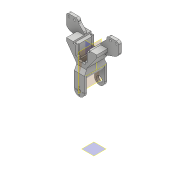
# Autodesk Inventor part: core_structure
Saved by Autodesk Inventor 2018 (Build 220112000, 112)
## iProperties
Created: 2018-02-12
Part Number: core_structure
Material: Generic
Document SubType Name: Modeling
Designer: Bardo91
Density: 1 g/cm^3
Appearance: Default
Author: Bardo91
Autodesk Inventor part; units mm, degrees
ref_plane "YZ Plane" through (0, 0, 0) normal (1, 0, 0) x (0, 1, 0)
ref_plane "XZ Plane" through (0, 0, 0) normal (0, 1, 0) x (-1, 0, 0)
ref_plane "XY Plane" through (0, 0, 0) normal (0, 0, 1) x (1, 0, 0)
sketch "Sketch1" plane through (0, 0, 0) normal (0, 0, 1) x (1, 0, 0)
  line L0 (0, 0) -> (18, 0)
  line L1 (18, 0) -> (18, 32)
  line L2 (18, 32) -> (0, 32)
  line L3 (0, 32) -> (0, 0)
  dimension "d0" = 18
  dimension "d1" = 32
  constraints: 8 end point, 2 perpendicular, 1 horizontal, 1 vertical
  measures "d0" distance of L0.start L0.end
  measures "d1" distance of L0.end L1.end
extrude "base" add sketch "Sketch1" along normal blind 25
sketch "Sketch2" plane through (0, 0, 25) normal (0, 0, 1) x (1, 0, 0)
  line L0 (18, 32) -> (0, 32) projected
  line L1 (9, 32) -> (9, 0)
  line L2 (9, 16) -> (9, 27.5)
  line L3 (9, 16) -> (20.5, 16) construction
  line L4 (9, 27.5) -> (15.25, 27.5)
  line L5 (15.25, 27.5) -> (15.25, 4.5)
  line L6 (15.25, 4.5) -> (2.75, 4.5)
  line L7 (2.75, 4.5) -> (2.75, 27.5)
  line L8 (2.75, 27.5) -> (9, 27.5)
  line L9 (0, 0) -> (18, 0) projected
  dimension "d4" = 11.5
  dimension "d5" = 90
  dimension "d6" = 6.25
  dimension "d7" = 23
  dimension "d8" = 12.5
  constraints: 16 end point, 6 perpendicular, 3 midpoint, 1 collinear, 1 horizontal, 1 point on line, 1 vertical
  measures "d4" distance of L2.start L2.end
  measures "d5" angle of L3 L2
  measures "d6" distance of L2.end L4.end
  measures "d7" distance of L4.end L5.end
  measures "d8" distance of L5.end L6.end
extrude "servo_place" cut sketch "Sketch2" against normal blind 18
sketch "Sketch3" plane through (0, 0, 25) normal (0, 0, 1) x (1, 0, 0)
  line L0 (2.75, 27.5) -> (15.25, 27.5) projected
  line L1 (9, 27.5) -> (9, 30.3)
  circle A0 centre (9, 30.3) radius 1
  line L2 (15.25, 4.5) -> (2.75, 4.5) projected
  line L3 (9, 4.5) -> (9, 1.7)
  circle A1 centre (9, 1.7) radius 1
  point P0 (0, 0)
  dimension "d11" = 2.8
  dimension "d12" = 2
  dimension "d13" = 2.8
  dimension "d14" = 2
  constraints: 4 end point, 2 centre point, 2 coincident, 2 midpoint, 2 vertical
  measures "d11" distance of L1.start L1.end
  measures "d12" diameter of A0
  measures "d13" distance of L3.start L3.end
  measures "d14" diameter of A1
extrude "screws_servo" cut sketch "Sketch3" against normal through all
ref_plane "Work Plane1" through (9, 22, -120) normal (0, 0, -1) x (-1, 0, 0)
sketch "Sketch6" plane through (0, 0, 25) normal (0, 0, 1) x (1, 0, 0)
  line L0 (0, 32) -> (0, 0) projected
  line L1 (2.75, 27.5) -> (15.25, 27.5) projected
  line L2 (0, 32) -> (2.75, 32)
  line L3 (2.75, 32) -> (2.75, 27.5)
  line L4 (2.75, 27.5) -> (0, 27.5)
  line L5 (0, 27.5) -> (0, 32)
  line L6 (18, 32) -> (15.2563, 32)
  line L7 (15.2563, 32) -> (15.2563, 27.5)
  line L8 (15.2563, 27.5) -> (18, 27.5)
  line L9 (18, 27.5) -> (18, 32)
  line L10 (15.25, 27.5) -> (15.25, 4.5) projected
  line L11 (18, 0) -> (15.25, 0)
  line L12 (15.25, 0) -> (15.25, 4.5)
  line L13 (15.25, 4.5) -> (18, 4.5)
  line L14 (18, 4.5) -> (18, 0)
  line L15 (0, 0) -> (2.75, 0)
  line L16 (2.75, 0) -> (2.75, 4.5)
  line L17 (2.75, 4.5) -> (0, 4.5)
  line L18 (0, 4.5) -> (0, 0)
  constraints: 32 end point, 8 parallel, 4 horizontal, 4 perpendicular, 4 point on line
extrude "pilars_top" add sketch "Sketch6" along normal blind 20
sketch "Sketch9" plane through (0, 0, 45) normal (0, 0, 1) x (1, 0, 0)
  line L0 (0, 32) -> (0, 0) projected
  line L1 (18, 0) -> (18, 32) projected
  line L2 (0, 32) -> (18, 32)
  line L3 (18, 32) -> (18, 0)
  line L4 (18, 0) -> (0, 0)
  line L5 (0, 0) -> (0, 32)
  line L6 (18, 32) -> (36, 32)
  line L7 (36, 32) -> (36, 0)
  line L8 (36, 0) -> (18, 0)
  line L9 (0, 32) -> (-18, 32)
  line L10 (-18, 32) -> (-18, 0)
  line L11 (-18, 0) -> (0, 0)
  point P0 (0, 22)
  point P1 (18, 22)
  dimension "d39" = 18
  dimension "d40" = 18
  constraints: 20 end point, 5 perpendicular, 3 parallel, 1 horizontal, 1 point on line, 1 vertical
  measures "d39" distance of L1.end L6.end
  measures "d40" distance of L0.start L9.end
extrude "base_top" add sketch "Sketch9" along normal blind 5
sketch "Sketch10" plane through (0, 0, 50) normal (0, 0, 1) x (1, 0, 0)
  line L0 (18, 32) -> (0, 32) projected
  line L1 (15.293, 32) -> (15.293, 0)
  line L2 (15.25, 27.5) -> (15.25, 4.5) projected
  line L3 (15.2563, 27.5) -> (15.2563, 32) projected
  line L4 (15.2563, 32) -> (2.7563, 32)
  line L5 (36, 32) -> (-18, 32) projected
  line L6 (2.7563, 32) -> (2.7563, 0)
  line L7 (0, 0) -> (18, 0) projected
  line L8 (15.293, 0) -> (2.7563, 0)
  dimension "d100" = 12.5
  constraints: 8 end point, 3 point on line, 1 collinear, 1 parallel, 1 perpendicular
  measures "d100" distance of L3.end L4.end
extrude "screw_hole" cut sketch "Sketch10" against normal blind 5
ref_plane "Work Plane2" through (0, 0, 10) normal (0, 0, -1) x (-1, 0, 0)
sketch "Sketch12" plane through (0, 0, 10) normal (0, 0, -1) x (-1, 0, 0)
  line L0 (0, 0) -> (-18, 0) projected
  line L1 (-18, 0) -> (-18, -4)
  line L2 (-18, -4) -> (0, -4)
  line L3 (0, -4) -> (0, 0)
  line L4 (0, 0) -> (0, -4)
  line L5 (0, 0) -> (-18, 0)
  line L6 (-18, 32) -> (0, 32) projected
  line L7 (-18, 32) -> (0, 32)
  line L8 (0, 32) -> (0, 36)
  line L9 (0, 36) -> (-18, 36)
  line L10 (-18, 36) -> (-18, 32)
  dimension "d64" = 4
  dimension "d65" = 4
  constraints: 18 end point, 4 perpendicular, 3 collinear, 2 point on line, 1 vertical
  measures "d64" distance of L0.end L1.end
  measures "d65" distance of L6.end L8.end
extrude "connector_prev_servo" add sketch "Sketch12" along normal blind 36
chamfer "Chamfer2" distance 8 distance2 4 1 edges at (9, 32, 10) measured on face at (9, 32, 10.5)
fillet "Fillet3" radius 9 4 edges at (18, 34, -26) (0, 34, -26) (0, -2, -26) (18, -2, -26)
sketch "Sketch13" plane through (0, -4, 10) normal (0, -1, 0) x (1, 0, 0)
  arc A0 (0, -27) -> (18, -27) centre (9, -27) ccw projected
  circle A1 centre (9, -27) radius 2.75
  line L0 (9, -27) -> (15, -27)
  circle A2 centre (15, -27) radius 1
  circle A3 centre (9, -21) radius 1
  circle A4 centre (3, -27) radius 1
  circle A5 centre (9, -33) radius 1
  point P0 (0, -10)
  dimension "d72" = 5.5
  dimension "d73" = 6
  dimension "d74" = 2
  dimension "d77" = 360
  constraints: 5 centre point, 2 coincident, 2 end point, 1 horizontal, 9 other
  measures "d72" diameter of A1
  measures "d73" distance of L0.start L0.end
  measures "d74" diameter of A2
extrude "screw_holes" cut sketch "Sketch13" against normal up to surface (4 mm away)
fillet "Fillet4" radius 9 2 edges at (18, 16, 0) (0, 16, 0)
sketch "Sketch14" plane through (0, 36, 10) normal (0, 1, 0) x (1, 0, 0)
  arc A0 (18, 27) -> (0, 27) centre (9, 27) ccw projected
  circle A1 centre (9, 27) radius 5.25
  point P0 (0, 10)
  dimension "d82" = 10.5
  constraints: 1 centre point, 1 coincident
  measures "d82" diameter of A1
extrude "Extrusion14" cut sketch "Sketch14" against normal up to next
sketch "Sketch16" plane through (2.75, 0, 25) normal (0, -1, 0) x (1, 0, 0)
  line L0 (12.5063, 20) -> (15.25, 20) projected
  line L1 (15.25, 20) -> (33.25, 20)
  line L2 (15.25, 20) -> (15.25, -5)
  line L3 (15.25, -7) -> (15.25, 20) projected
  line L4 (15.25, -5) -> (33.25, 20)
  point P0 (-2.75, -25)
  dimension "d95" = 25
  constraints: 6 end point, 1 horizontal, 1 point on line
  measures "d95" distance of L0.end L2.end
extrude "Extrusion16" add sketch "Sketch16" against normal blind 4.6
ref_plane "Work Plane3" through (2.75, 16, 25) normal (0, 1, 0) x (1, 0, 0)
ref_plane "Work Plane4" through (9, -4, -17) normal (1, 0, 0) x (0, 0, -1)
mirror "Mirror1" about plane through (2.75, 16, 25) normal (0, 1, 0) of "Extrusion16"
mirror "Mirror2" about plane through (9, -4, -17) normal (1, 0, 0) of "Extrusion16", "Mirror1"
sketch "Sketch18" plane through (2.75, 0, 25) normal (0, -1, 0) x (1, 0, 0)
  line L0 (12.5, 0) -> (0, 0) projected
  line L1 (6.25, 0) -> (6.25, 5)
  line L2 (6.25, 5) -> (-3.75, 5)
  line L3 (-3.75, 5) -> (-3.75, 25)
  line L4 (-20.75, 25) -> (0.0063, 25) projected
  line L5 (-3.75, 25) -> (16.25, 25)
  line L6 (16.25, 25) -> (16.25, 5)
  line L7 (16.25, 5) -> (6.25, 5)
  point P0 (-2.75, -25)
  dimension "d105" = 5
  dimension "d106" = 10
  dimension "d107" = 20
  constraints: 12 end point, 5 perpendicular, 2 point on line, 1 midpoint, 1 vertical
  measures "d105" distance of L1.start L1.end
  measures "d106" distance of L1.end L2.end
  measures "d107" distance of L3.end L5.end
extrude "Extrusion18" cut sketch "Sketch18" against normal through all
sketch "Sketch19" plane through (0, 0, 50) normal (0, 0, 1) x (1, 0, 0)
  line L0 (-1, 0) -> (-1, 32) projected
  line L1 (-1, 32) -> (-6, 32)
  line L2 (0, 32) -> (-18, 32) projected
  line L3 (-6, 32) -> (-6, 0)
  line L4 (-6, 0) -> (24, 0)
  line L5 (24, 0) -> (24, 32)
  line L6 (24, 32) -> (-1, 32)
  point P0 (0, 0)
  dimension "d110" = 5
  dimension "d111" = 30
  constraints: 10 end point, 4 perpendicular, 2 point on line
  measures "d110" distance of L0.end L1.end
  measures "d111" distance of L3.end L4.end
extrude "Extrusion19" cut sketch "Sketch19" against normal blind 3
sketch "Sketch20" plane through (0, 0, 47) normal (0, 0, 1) x (1, 0, 0)
  line L0 (-6, 32) -> (-1, 32) projected
  line L1 (-6, 32) -> (-3.5, 32)
  line L2 (-3.5, 32) -> (-3.5, 29.5)
  circle A0 centre (-3.5, 29.5) radius 1.4
  point P0 (0, 0)
  dimension "d114" = 2.5
  dimension "d115" = 2.5
  dimension "d116" = 2.8
  constraints: 4 end point, 1 centre point, 1 coincident, 1 midpoint, 1 perpendicular
  measures "d114" distance of L0.start L1.end
  measures "d115" distance of L1.end L2.end
  measures "d116" diameter of A0
extrude "Extrusion20" cut sketch "Sketch20" against normal blind 5
mirror "Mirror3" about plane through (9, -4, -17) normal (1, 0, 0) of "Extrusion20"
mirror "Mirror4" about plane through (2.75, 16, 25) normal (0, 1, 0) of "Extrusion20", "Mirror3"
sketch "Sketch21" plane through (0, 0, 25) normal (0, 0, 1) x (1, 0, 0)
  line L0 (2.75, 4.5) -> (2.75, 27.5) projected
  line L1 (2.75, 16) -> (2.75, 27.75)
  line L2 (2.75, 27.75) -> (15.25, 27.75)
  line L3 (15.25, 27.75) -> (15.25, 4.25)
  line L4 (15.25, 27.5) -> (15.25, 4.5) projected
  line L5 (15.25, 4.25) -> (2.75, 4.25)
  line L6 (2.75, 4.25) -> (2.75, 16)
  point P0 (0, 0)
  dimension "d119" = 11.75
  dimension "d120" = 12.5
  dimension "d121" = 23.5
  dimension "d122" = 12.5
  constraints: 10 end point, 2 collinear, 1 midpoint, 1 perpendicular, 1 point on line
  measures "d119" distance of L1.start L1.end
  measures "d120" distance of L1.end L2.end
  measures "d121" distance of L2.end L3.end
  measures "d122" distance of L3.end L5.end
extrude "Extrusion21" cut sketch "Sketch21" against normal up to surface (18 mm away)
sketch "Sketch22" plane through (2.75, 27.75, 25) normal (0, -1, 0) x (1, 0, 0)
  line L0 (12.5, 0) -> (12.5, -18) projected
  line L1 (0, -18) -> (12.5, -18) projected
  line L2 (12.5, -18) -> (0, -18)
  line L3 (0, -18) -> (0, -11)
  line L4 (0, -11) -> (12.5, -11)
  line L5 (12.5, -11) -> (12.5, -18)
  point P0 (-2.75, -25)
  dimension "d125" = 7
  constraints: 8 end point, 3 perpendicular, 1 collinear
  measures "d125" distance of L1.start L3.end
extrude "Extrusion22" cut sketch "Sketch22" against normal through all
chamfer "Chamfer3" distance 8 distance2 4 1 edges at (9, 0, 10) measured on face at (9, 0, 10.5)
sketch "Sketch23" plane through (18, 27.4, 20) normal (0, -1, 0) x (1, 0, 0)
  line L0 (18, 25) -> (1, 25) projected
  line L1 (18, 25) -> (1, 25)
  line L2 (0, 0) -> (18, 25) projected
  line L3 (18, 25) -> (0, 0)
  line L4 (0, 0) -> (0, 5) projected
  line L5 (0, 0) -> (0, 27)
  line L6 (0, 27) -> (18, 27)
  line L7 (18, 27) -> (18, 25)
  line L8 (-35.987, 24.982) -> (-18, 0)
  line L9 (-18, 0) -> (-36, 25) projected
  line L10 (-18, 0) -> (-18, 27)
  line L11 (-18, 27) -> (-35.987, 27)
  line L12 (-35.987, 27) -> (-35.987, 24.982)
  point P0 (-18, -20)
  dimension "d131" = 27
  dimension "d132" = 27
  constraints: 18 end point, 4 perpendicular, 3 collinear, 2 point on line, 1 horizontal, 1 vertical
  measures "d131" distance of L5.start L5.end
  measures "d132" distance of L8.end L10.end
extrude "Extrusion23" add sketch "Sketch23" along normal up to surface (22.8 mm away)
sketch "Sketch11" plane through (0, 0, 50) normal (0, 0, 1) x (1, 0, 0)
  circle A0 centre (9, 22) radius 6 projected
  line L0 (9, 22) -> (36, 22)
  line L1 (36, 0) -> (36, 32) projected
  line L2 (36, 22) -> (36, 24.5)
  line L3 (36, 24.5) -> (31, 24.5)
  line L4 (31, 24.5) -> (31, 19.5)
  line L5 (31, 19.5) -> (36, 19.5)
  line L6 (36, 19.5) -> (36, 24.5)
  line L7 (9, 22) -> (9, 34.0709)
  line L8 (-18, 22) -> (-18, 24.5)
  line L9 (-18, 24.5) -> (-13, 24.5)
  line L10 (-13, 24.5) -> (-13, 19.5)
  line L11 (-13, 19.5) -> (-18, 19.5)
  line L12 (-18, 19.5) -> (-18, 24.5)
  dimension "d60" = 2.5
  dimension "d61" = 5
  dimension "d62" = 5
  constraints: 24 end point, 5 symmetric about line, 3 perpendicular, 3 point on line, 1 collinear, 1 horizontal, 1 vertical
  measures "d60" distance of L0.end L2.end
  measures "d61" distance of L2.end L3.end
  measures "d62" distance of L3.end L4.end
extrude "Extrusion11" cut sketch "Sketch11" against normal through all contours L4 L3 L1 L0 | L0 L1 L5 L4 | L8 L9 L10 L11 L12
sketch "Sketch24" plane through (31, 19.5, 50) normal (0, 1, 0) x (1, 0, 0)
  line L0 (0, 0) -> (10, 0)
  line L1 (0, 0) -> (5, 0) projected
  line L2 (10, 0) -> (10, -15)
  circle A0 centre (10, -15) radius 1.75
  line L3 (10, -15) -> (20, -15)
  circle A1 centre (20, -15) radius 1.75
  line L4 (-7, 0) -> (5, 0) projected
  line L5 (-7, 0) -> (-7, -3)
  line L6 (-7, -3) -> (3.6066, -13.6066)
  line L7 (3.6066, -13.6066) -> (3.6066, -19.6066)
  line L8 (3.6066, -19.6066) -> (24.6066, -19.6066)
  line L9 (24.6066, -19.6066) -> (24.6066, 0.3934)
  line L10 (24.6066, 0.3934) -> (20.364, 4.636)
  line L11 (5, 5) -> (5, 0) projected
  line L12 (0, 4.636) -> (0, 0)
  line L13 (5, 5) -> (0, 11.9444) projected
  line L14 (20.364, 4.636) -> (0, 11.9444)
  line L15 (0, 11.9444) -> (0, 4.636)
  point P0 (-31, 50)
  dimension "d135" = 10
  dimension "d136" = 15
  dimension "d137" = 3.5
  dimension "d138" = 10
  dimension "d139" = 3.5
  dimension "d140" = 3
  dimension "d141" = 15
  dimension "d142" = 135
  dimension "d143" = 6
  dimension "d144" = 21
  dimension "d145" = 20
  dimension "d146" = 6
  constraints: 24 end point, 2 centre point, 2 coincident, 2 collinear, 2 parallel, 2 perpendicular, 2 vertical, 1 horizontal
  measures "d135" distance of L0.start L0.end
  measures "d136" distance of L0.end L2.end
  measures "d137" diameter of A0
  measures "d138" distance of L3.start L3.end
  measures "d139" diameter of A1
  measures "d140" distance of L4.start L5.end
  measures "d141" distance of L5.end L6.end
  measures "d142" angle of L6 L5
  measures "d143" distance of L6.end L7.end
  measures "d144" distance of L7.end L8.end
  measures "d145" distance of L8.end L9.end
  measures "d146" distance of L9.end L10.end
extrude "Extrusion24" add sketch "Sketch24" along normal blind 5 contours L0 L11 L13 L14 L10 L9 L8 L7 L6 L5 L4
fillet "Fillet5" radius 4 6 edges at (55.6066, 22, 69.6066) (34.6066, 22, 69.6066) (34.6066, 22, 63.6066) (55.6066, 22, 49.6066) (51.364, 22, 45.364) (24, 22, 53)
mirror "Mirror5" about plane through (9, -4, -17) normal (1, 0, 0) of "Extrusion24", "Fillet5"
sketch "Sketch25" plane through (0, 0, 25) normal (0, 0, 1) x (1, 0, 0)
  line L0 (2.75, 4.5) -> (2.75, 27.5) projected
  line L1 (2.75, 16) -> (2.75, 3.5)
  line L2 (2.75, 3.5) -> (15.25, 3.5)
  line L3 (15.25, 4.25) -> (2.75, 4.25) projected
  line L4 (15.25, 3.5) -> (15.25, 28.5)
  line L5 (15.25, 27.75) -> (15.25, 4.5) projected
  line L6 (15.25, 28.5) -> (2.75, 28.5)
  line L7 (2.75, 28.5) -> (2.75, 16)
  point P0 (0, 0)
  dimension "d150" = 12.5
  dimension "d151" = 25
  constraints: 10 end point, 3 collinear, 1 midpoint, 1 parallel, 1 perpendicular, 1 point on line
  measures "d150" distance of L1.start L1.end
  measures "d151" distance of L2.end L4.end
extrude "Extrusion25" cut sketch "Sketch25" against normal up to surface (18 mm away)
equation "\"d151\" = 2 * d150"
body "Solid1"
